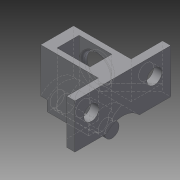
# Autodesk Inventor part: chain_end_2020
Saved by Autodesk Inventor 2014 (Build 180170000, 170)
## iProperties
Created: 2016-05-16
Part Number: chain_end_2020
Material: Generic
Document SubType Name: Modeling
Designer: 101767
Density: 1 g/cm^3
Appearance: Default
Author: 101767
Autodesk Inventor part; units mm, degrees
ref_plane "YZ Plane" through (0, 0, 0) normal (1, 0, 0) x (0, 1, 0)
sketch "Sketch1" plane through (0, 0, 0) normal (0, 0, 1) x (1, 0, 0)
  line L0 (0, 0) -> (15.2, 0)
  line L1 (15.2, 0) -> (15.2, 12)
  line L2 (15.2, 12) -> (0, 12)
  line L3 (0, 12) -> (0, 0)
  line L4 (1.6, 10) -> (13.6, 10)
  line L5 (13.6, 10) -> (13.6, 2)
  line L6 (13.6, 2) -> (1.6, 2)
  line L7 (1.6, 2) -> (1.6, 10)
  dimension "d0" = 15.2
  dimension "d1" = 12
  dimension "d2" = 1.6
  dimension "d3" = 2
  dimension "d4" = 2
  dimension "d5" = 1.6
  constraints: 16 end point, 4 parallel, 2 horizontal, 2 perpendicular
  measures "d0" distance of L1.end L2.end
  measures "d1" distance of L0.end L1.end
  measures "d2" distance between parallel lines of L3 L7
  measures "d3" distance between parallel lines of L2 L4
  measures "d4" distance between parallel lines of L0 L6
  measures "d5" distance between parallel lines of L1 L5
extrude "Extrusion1" add sketch "Sketch1" along normal blind 20
sketch "Sketch2" plane through (0, 0, 0) normal (1, 0, 0) x (0, 1, 0)
  line L0 (0, 0) -> (12, 0) construction
  line L1 (6, 13.0663) -> (6, -2.0093) construction
  line L2 (0, 0) -> (0, 20) construction
  line L3 (12, 0) -> (12, 20) construction
  line L4 (6, 0) -> (12, 3.8224)
  line L5 (12, 3.8224) -> (12, 0)
  line L6 (12, 0) -> (6, 0)
  dimension "d8" = 12
  dimension "d9" = 6
  dimension "d10" = 32.5
  constraints: 8 end point, 2 collinear, 2 point on line, 1 midpoint, 1 perpendicular
  measures "d8" distance of L0.start L0.end
  measures "d9" distance between parallel lines of L2 L1
  measures "d10" angle of L0 L4
extrude "Extrusion2" cut sketch "Sketch2" along normal through all
sketch "Sketch4" plane through (1.6, 2, 20) normal (1, 0, 0) x (0, 0, -1)
  circle A0 centre (20, 4) radius 2.6
  point P0 (20, -2)
  dimension "d14" = 5.2
  constraints: 1 centre point, 1 coincident
  measures "d14" diameter of A0
extrude "Extrusion3" add sketch "Sketch4" against normal blind 4
sketch "Sketch5" plane through (0, 0, 20) normal (-1, 0, 0) x (0, 0, 1)
  line L0 (-20, 0) -> (0, 0) construction
  line L1 (0, 12) -> (0, 0) construction
  line L2 (-16.1776, 12) -> (0, 12) construction
  arc A0 (-16.1776, 0) -> (-16.1776, 12) centre (-21.4691, 6) ccw
  line L3 (-16.1776, 12) -> (0, 12)
  line L4 (0, 0) -> (-16.1776, 0)
  line L5 (0, 0) -> (0, 12)
  dimension "d17" = 8
  constraints: 6 end point, 3 collinear, 2 point on circle, 1 centre point, 1 point on line, 1 vertical alignment
  measures "d17" radius of A0
extrude "Extrusion4" add sketch "Sketch5" along normal blind 2.4
ref_plane "Work Plane2" through (7.6, 2, 20) normal (1, 0, 0) x (0, 0, -1)
mirror "Mirror1" about plane through (7.6, 2, 20) normal (1, 0, 0) of "Extrusion3", "Extrusion4"
fillet "Fillet1" radius 2 4 edges at (14.4, 8.1928, 1.397) (0.8, 8.1928, 1.397) (14.4, 3.4, 0) (0.8, 3.4, 0)
sketch "Sketch9" plane through (17.6, 6, -1.4691) normal (1, 0, 0) x (0, 0, -1)
  line L0 (-5.2915, -6) -> (-21.4691, -6) projected
  arc A0 (-5.2915, 6) -> (-5.2915, -6) centre (0, 0) ccw projected
  line L1 (-21.4691, 6) -> (-5.2915, 6) projected
  line L2 (-21.4691, -6) -> (-21.4691, 6) projected
  point P0 (-1.4691, -6)
extrude "Extrusion8" add sketch "Sketch9" along normal blind 1
sketch "Sketch10" plane through (18.6, 6, -1.4691) normal (1, 0, 0) x (0, 0, -1)
  arc A0 (-5.2915, 6) -> (-5.2915, -6) centre (0, 0) ccw construction
  line L0 (-21.4691, 6) -> (-21.4691, -6) construction
  line L1 (-21.4691, 17.5) -> (-8, 17.5)
  line L2 (-8, 17.5) -> (-8, -17.5)
  line L3 (-8, -17.5) -> (-21.4691, -17.5)
  line L4 (-21.4691, -17.5) -> (-21.4691, 17.5)
  line L5 (0, 0) -> (-40.6446, 0) construction
  line L6 (-5.2915, 6) -> (-21.4691, 6) construction
  circle A1 centre (-14.7345, 11.5) radius 2.75
  line L7 (-14.7345, 17.5) -> (-14.7345, -17.5) construction
  circle A2 centre (-14.7345, -11.5) radius 2.75
  dimension "d37" = 35
  dimension "d38" = 17.5
  dimension "d41" = 5.5
  dimension "d42" = 5.5
  constraints: 12 end point, 2 centre point, 2 midpoint, 2 parallel, 2 perpendicular, 1 collinear, 1 horizontal, 1 point on line, 1 symmetric about line, 1 tangent, 1 other
  measures "d37" distance of L3.end L1.start
  measures "d38" distance between parallel lines of L5 L3
  measures "d41" diameter of A1
  measures "d42" distance from line of L6 A1.centre
extrude "Extrusion10" add sketch "Sketch10" along normal blind 3
sketch "Sketch11" plane through (18.6, 12, 6.5309) normal (0, 0, -1) x (-1, 0, 0)
  line L0 (0, -23.5) -> (-3, -23.5) construction
  line L1 (0, -12) -> (0, -23.5) construction
  line L2 (18.6, -12) -> (3.4, -12) construction
  line L3 (-3, -12) -> (11.5, -12)
  line L4 (11.5, -12) -> (0, -23.5)
  line L5 (0, -23.5) -> (-3, -23.5)
  line L6 (-3, -12) -> (-3, -23.5)
  dimension "d47" = 45
  constraints: 8 end point, 2 collinear, 1 perpendicular, 1 point on line
  measures "d47" angle of L1 L4
extrude "Extrusion11" add sketch "Sketch11" along normal up to surface (2.7085 mm away)
ref_plane "Work Plane4" through (1.6, 6, 20) normal (0, 1, 0) x (1, 0, 0)
mirror "Mirror3" about plane through (1.6, 6, 20) normal (0, 1, 0) of "Extrusion11"
sketch "Sketch13" plane through (21.6, 6, -1.4691) normal (1, 0, 0) x (0, 0, -1)
  line L0 (-8, -6) -> (-5.2915, -6) projected
  line L1 (-8, -6) -> (-8, 6) projected
  line L2 (-8, 6) -> (-5.2915, 6) projected
  arc A0 (-5.2915, 6) -> (-8, 0) centre (0, 0) ccw projected
  arc A1 (-8, 0) -> (-5.2915, -6) centre (0, 0) ccw projected
  point P0 (-1.4691, -6)
extrude "Extrusion13" add sketch "Sketch13" against normal up to surface (3 mm away)
sketch "Sketch14" plane through (-2.4, 12, 3.8224) normal (0, 1, 0) x (1, 0, 0)
  line L0 (4, 1.2741) -> (4, -16.1776) construction
  line L1 (16, 1.2741) -> (16, -16.1776) construction
  line L2 (9.5, 0) -> (2.4, 0) construction
  line L3 (0, -16.1776) -> (21, -16.1776) construction
  circle A0 centre (10, -8.1776) radius 5
  dimension "d54" = 10
  dimension "d56" = 12
  dimension "d57" = 6
  dimension "d58" = 8
  constraints: 1 centre point
  measures "d54" diameter of A0
  measures "d56" distance between parallel lines of L1 L0
  measures "d57" distance from line of L0 A0.centre
  measures "d58" distance from line of A0.centre L3
extrude "Extrusion14" cut sketch "Sketch14" against normal blind 3
fillet "Fillet2" radius 1 1 edges at (2.6, 10, 12)
equation "\"d9\" = 0.5 * d8"
equation "\"d38\" = 0.5 * d37"
equation "\"d57\" = 0.5 * d56"
body "Solid1"
